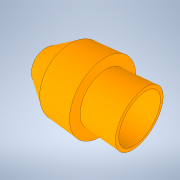
# Autodesk Inventor part: Сопло для воды
Saved by Autodesk Inventor 2021.1 (Build 251245010, 245A)
## iProperties
Created: 2026-04-21
Part Number: Сопло для воды
Material: Типовые
Document SubType Name: Modeling
Designer: Андрей Тарасов
Density: 1 g/cm^3
Appearance: По умолчанию
Author: Андрей Тарасов
Autodesk Inventor part; units mm, degrees
ref_plane "YZ Plane" through (0, 0, 0) normal (1, 0, 0) x (0, 1, 0)
ref_plane "XZ Plane" through (0, 0, 0) normal (0, 1, 0) x (-1, 0, 0)
ref_plane "XY Plane" through (0, 0, 0) normal (0, 0, 1) x (1, 0, 0)
sketch "Эскиз2" plane through (0, 0, 0) normal (0, 0, 1) x (1, 0, 0)
  line L0 (0, 1) -> (0, 3)
  line L1 (0, 3) -> (5, 5.5)
  line L2 (5, 5.5) -> (10, 5.5)
  line L3 (10, 5.5) -> (10, 3.5)
  line L4 (-3, 0) -> (18, 0) construction
  line L5 (0, 1) -> (4, 1)
  line L6 (4, 1) -> (4, 2.8)
  line L7 (4, 2.8) -> (4.7, 3.5)
  line L8 (4.7, 3.5) -> (10, 3.5)
  line L9 (4, 1) -> (6, 1)
  line L10 (6, 1) -> (6, 1.4)
  line L11 (6, 1.4) -> (4, 1.4)
  line L12 (10, 3.5) -> (15, 3.5)
  line L13 (15, 3.5) -> (15, 4)
  line L14 (15, 4) -> (10, 4)
  point P0 (0, 0)
  point P1 (3.6, 3)
  point P2 (10, 4)
  dimension "d6" = 2
  dimension "d7" = 5
  dimension "d10" = 4
  dimension "d12" = 2.5
  dimension "d13" = 1
  dimension "d14" = 1.8
  dimension "d15" = 10
  dimension "d27" = 0.4
  dimension "d28" = 2
  dimension "d34" = 135
  dimension "d35" = 0.5
  dimension "d36" = 5
  dimension "d37" = 2
  constraints: 28 end point, 6 perpendicular, 4 horizontal, 3 point on line, 1 parallel
  measures "d6" distance of L0.start L0.end
  measures "d7" distance of L1.end L2.end
  measures "d10" distance of L0.start L5.end
  measures "d12" distance between parallel lines of L8 L5
  measures "d13" distance between parallel lines of L4 L5
  measures "d14" distance of L5.end L6.end
  measures "d15" distance between parallel lines of L3 L0
  measures "d27" distance between parallel lines of L9 L11
  measures "d28" distance between parallel lines of L6 L10
  measures "d34" angle of L6 L7
  measures "d35" distance of L12.end L13.end
  measures "d36" distance between parallel lines of L3 L13
  measures "d37" distance between parallel lines of L8 L2
revolve "Вращение1" add sketch "Эскиз2" angle 360 about axis through (-10, 0, 0) along (1, 0, 0)
chamfer "Фаска2" distance 0.6 angle 45 1 edges at (4, -1.4, 0)
